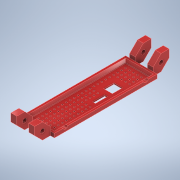
# Autodesk Inventor part: Prod05.3.2 - SKR1.4 Turbo Case Front
Saved by Autodesk Inventor 2021 (Build 250183000, 183)
## iProperties
Created: 2021-06-22
Part Number: Prod05.3.2 - SKR1.4 Turbo Case Front
Material: Generic
Document SubType Name: Modeling
Designer: alexr
Density: 1 g/cm^3
Appearance: Red
Author: alexr
Autodesk Inventor part; units mm, degrees
ref_plane "YZ Plane" through (0, 0, 0) normal (1, 0, 0) x (0, 1, 0)
ref_plane "XZ Plane" through (0, 0, 0) normal (0, 1, 0) x (-1, 0, 0)
ref_plane "XY Plane" through (0, 0, 0) normal (0, 0, 1) x (1, 0, 0)
sketch "Base Profile" plane through (0, 0, 0) normal (1, 0, 0) x (0, 1, 0)
  line L0 (10, 0) -> (20, 0)
  line L1 (20, 0) -> (20, -10)
  line L2 (10, -20) -> (5, -20)
  line L3 (0, -20) -> (0, -10)
  line L4 (0, -20) -> (0, -150)
  line L5 (5, -20) -> (5, -150)
  line L6 (5, -150) -> (10, -150)
  line L7 (20, -160) -> (20, -170)
  line L8 (20, -170) -> (10, -170)
  line L9 (0, -160) -> (0, -150)
  line L10 (0, -160) -> (10, -170)
  line L11 (10, 0) -> (0, -10)
  line L12 (20, -10) -> (10, -20)
  line L13 (10, -150) -> (20, -160)
  point P0 (0, 0)
  point P1 (20, -20)
  point P2 (10, -10)
  point P3 (20, -150)
  point P4 (0, -170)
  point P5 (10, -160)
  dimension "d0" = 20
  dimension "d1" = 20
  dimension "d3" = 130
  dimension "d4" = 5
  dimension "d5" = 20
  dimension "d6" = 20
  constraints: 28 end point, 8 point on line, 5 parallel, 2 horizontal, 2 perpendicular, 1 vertical
  measures "d0" distance of point (20, -20) L3.start
  measures "d1" distance of L0.end point (20, -20)
  measures "d3" distance of L3.start L4.end
  measures "d4" distance between parallel lines of L4 L5
  measures "d5" distance of L7.end point (0, -170)
  measures "d6" distance of point (20, -150) L7.end
extrude "Base Extrusion" add sketch "Base Profile" along normal blind 40
hole "Fixing Holes" at (0, 10, -160) at (0, 10, -10) direction (1, 0, 0) diameter 5.5 end through all
sketch "Cutouts" plane through (0, 0, -160) normal (0, -1, 0) x (1, 0, 0)
  line L0 (0, 10) -> (40, 10) projected
  line L1 (0, 10) -> (5.1, 10)
  line L2 (5.1, 10) -> (5.1, -10)
  line L3 (5.1, -10) -> (0, -10)
  line L4 (0, -10) -> (0, 10)
  line L5 (40, -10) -> (40, 0) projected
  line L6 (40, -10) -> (34.9, -10)
  line L7 (34.9, -10) -> (34.9, 10)
  line L8 (34.9, 10) -> (40, 10)
  line L9 (40, 10) -> (40, -10)
  line L10 (40, 160) -> (40, 150) projected
  line L11 (40, 160) -> (34.9, 160)
  line L12 (34.9, 160) -> (34.9, 140)
  line L13 (34.9, 140) -> (40, 140)
  line L14 (40, 140) -> (40, 160)
  line L15 (0, 160) -> (5.1, 160)
  line L16 (5.1, 160) -> (5.1, 140)
  line L17 (5.1, 140) -> (0, 140)
  line L18 (0, 140) -> (0, 160)
  line L19 (18.75, 43.5) -> (29.75, 43.5)
  line L20 (29.75, 43.5) -> (29.75, 56.5)
  line L21 (29.75, 56.5) -> (18.75, 56.5)
  line L22 (18.75, 56.5) -> (18.75, 43.5)
  line L23 (40, 150) -> (40, 0) projected
  line L24 (0, -10) -> (40, -10) projected
  line L25 (26, 62.5) -> (29.75, 62.5)
  line L26 (29.75, 62.5) -> (29.75, 78)
  line L27 (29.75, 78) -> (26, 78)
  line L28 (26, 78) -> (26, 62.5)
  line L29 (12.4, -10) -> (27.6, -10)
  line L30 (27.6, -10) -> (27.6, 10)
  line L31 (27.6, 10) -> (12.4, 10)
  line L32 (12.4, 10) -> (12.4, -10)
  line L33 (0, 160) -> (40, 160) projected
  line L34 (12.4, 160) -> (27.6, 160)
  line L35 (27.6, 160) -> (27.6, 140)
  line L36 (27.6, 140) -> (12.4, 140)
  line L37 (12.4, 140) -> (12.4, 160)
  line L38 (35, 95) -> (35, 125) construction
  line L39 (5, 125) -> (5, 95) construction
  line L40 (0, 150) -> (0, 0) projected
  point P0 (34.9, 10)
  point P1 (12.4, 10)
  point P2 (27.6, 10)
  point P3 (5, 20)
  point P4 (5, 25)
  point P5 (5, 30)
  point P6 (5, 35)
  point P7 (5, 40)
  point P8 (5, 45)
  point P9 (5, 50)
  point P10 (5, 55)
  point P11 (5, 60)
  point P12 (5, 65)
  point P13 (5, 70)
  point P14 (5, 75)
  point P15 (5, 80)
  point P16 (5, 85)
  point P17 (5, 90)
  point P18 (5, 95)
  point P19 (5, 100)
  point P20 (5, 105)
  point P21 (5, 110)
  point P22 (5, 115)
  point P23 (5, 120)
  point P24 (5, 125)
  point P25 (5, 130)
  point P26 (10, 20)
  point P27 (10, 25)
  point P28 (10, 30)
  point P29 (10, 35)
  point P30 (10, 40)
  point P31 (10, 45)
  point P32 (10, 50)
  point P33 (10, 55)
  point P34 (10, 60)
  point P35 (10, 65)
  point P36 (10, 70)
  point P37 (10, 75)
  point P38 (10, 80)
  point P39 (10, 85)
  point P40 (10, 90)
  point P41 (10, 95)
  point P42 (10, 100)
  point P43 (10, 105)
  point P44 (10, 110)
  point P45 (10, 115)
  point P46 (10, 120)
  point P47 (10, 125)
  point P48 (10, 130)
  point P49 (15, 20)
  point P50 (15, 25)
  point P51 (15, 30)
  point P52 (15, 35)
  point P53 (15, 40)
  point P54 (15, 45)
  point P55 (15, 50)
  point P56 (15, 55)
  point P57 (15, 60)
  point P58 (15, 65)
  point P59 (15, 70)
  point P60 (15, 75)
  point P61 (15, 80)
  point P62 (15, 85)
  point P63 (15, 90)
  point P64 (15, 95)
  point P65 (15, 100)
  point P66 (15, 105)
  point P67 (15, 110)
  point P68 (15, 115)
  point P69 (15, 120)
  point P70 (15, 125)
  point P71 (15, 130)
  point P72 (20, 20)
  point P73 (20, 25)
  point P74 (20, 30)
  point P75 (20, 35)
  point P76 (20, 40)
  point P77 (20, 45)
  point P78 (20, 50)
  point P79 (20, 55)
  point P80 (20, 60)
  point P81 (20, 65)
  point P82 (20, 70)
  point P83 (20, 75)
  point P84 (20, 80)
  point P85 (20, 85)
  point P86 (20, 90)
  point P87 (20, 95)
  point P88 (20, 100)
  point P89 (20, 105)
  point P90 (20, 110)
  point P91 (20, 115)
  point P92 (20, 120)
  point P93 (20, 125)
  point P94 (20, 130)
  point P95 (25, 20)
  point P96 (25, 25)
  point P97 (25, 30)
  point P98 (25, 35)
  point P99 (25, 40)
  point P100 (25, 45)
  point P101 (25, 50)
  point P102 (25, 55)
  point P103 (25, 60)
  point P104 (25, 65)
  point P105 (25, 70)
  point P106 (25, 75)
  point P107 (25, 80)
  point P108 (25, 85)
  point P109 (25, 90)
  point P110 (25, 95)
  point P111 (25, 100)
  point P112 (25, 105)
  point P113 (25, 110)
  point P114 (25, 115)
  point P115 (25, 120)
  point P116 (25, 125)
  point P117 (25, 130)
  point P118 (30, 20)
  point P119 (30, 25)
  point P120 (30, 30)
  point P121 (30, 35)
  point P122 (30, 40)
  point P123 (30, 45)
  point P124 (30, 50)
  point P125 (30, 55)
  point P126 (30, 60)
  point P127 (30, 65)
  point P128 (30, 70)
  point P129 (30, 75)
  point P130 (30, 80)
  point P131 (30, 85)
  point P132 (30, 90)
  point P133 (30, 95)
  point P134 (30, 100)
  point P135 (30, 105)
  point P136 (30, 110)
  point P137 (30, 115)
  point P138 (30, 120)
  point P139 (30, 125)
  point P140 (30, 130)
  point P141 (35, 20)
  point P142 (35, 25)
  point P143 (35, 30)
  point P144 (35, 35)
  point P145 (35, 40)
  point P146 (35, 45)
  point P147 (35, 50)
  point P148 (35, 55)
  point P149 (35, 60)
  point P150 (35, 65)
  point P151 (35, 70)
  point P152 (35, 75)
  point P153 (35, 80)
  point P154 (35, 85)
  point P155 (35, 90)
  point P156 (35, 95)
  point P157 (35, 100)
  point P158 (35, 105)
  point P159 (35, 110)
  point P160 (35, 115)
  point P161 (35, 120)
  point P162 (35, 125)
  point P163 (35, 130)
  dimension "d18" = 5.1
  dimension "d20" = 5.1
  dimension "d21" = 20
  dimension "d22" = 5.1
  dimension "d23" = 20
  dimension "d24" = 5.1
  dimension "d25" = 20
  dimension "d27" = 53.5
  dimension "d33" = 15.5
  dimension "d34" = 6
  dimension "d36" = 15.2
  dimension "d37" = 20
  dimension "d38" = 15.2
  dimension "d39" = 20
  dimension "d40" = 7.3
  dimension "d41" = 7.3
  dimension "d44" = 30
  dimension "d45" = 30
  dimension "d47" = 5
  dimension "d110" = 5
  dimension "d111" = 10.25
  dimension "d112" = 10.25
  dimension "d113" = 14
  dimension "d115" = 82
  dimension "d116" = 0
  dimension "d117" = 10
  dimension "d118" = 0
  dimension "d119" = 150
  dimension "d120" = 0
  dimension "d121" = 160
  dimension "d122" = 35
  dimension "d123" = 5.1
  dimension "d124" = 150
  dimension "d125" = 12.4
  dimension "d126" = 0
  dimension "d127" = 12.4
  dimension "d128" = 150
  dimension "d129" = 12.4
  dimension "d130" = 170
  dimension "d131" = 27.6
  dimension "d132" = 150
  dimension "d133" = 34.9
  dimension "d134" = 150
  dimension "d135" = 65
  dimension "d136" = 11
  dimension "d146" = 5
  dimension "d147" = 10
  dimension "d150" = 5
  dimension "d153" = 5
  constraints: 68 end point, 17 parallel, 9 horizontal, 8 perpendicular, 2 point on line, 1 vertical, 160 other
  measures "d18" distance of L2.end L3.end
  measures "d20" distance of L7.end L8.end
  measures "d21" distance of L6.end L7.end
  measures "d22" distance of L13.end L12.end
  measures "d23" distance of L12.end L11.end
  measures "d24" distance of L16.end L17.end
  measures "d25" distance of L15.end L16.end
  measures "d27" distance between parallel lines of L24 L19
  measures "d33" distance of L26.end L25.end
  measures "d34" distance between parallel lines of L21 L25
  measures "d36" distance of L31.end L30.end
  measures "d37" distance of L30.end L29.end
  measures "d38" distance of L35.end L36.end
  measures "d39" distance of L34.end L35.end
  measures "d40" distance between parallel lines of L12 L35
  measures "d41" distance between parallel lines of L30 L7
  measures "d44" distance of L39.start L38.end
  measures "d45" distance of L38.end L38.start
  measures "d47" distance between parallel lines of L40 L39
  measures "d110" distance between parallel lines of L10 L38
  measures "d111" distance between parallel lines of L10 L26
  measures "d112" distance between parallel lines of L10 L20
  measures "d113" distance between parallel lines of L10 L28
  measures "d115" distance between parallel lines of L27 L33
  measures "d116" distance from line of point (40, 150) L5
  measures "d117" distance from line of point (40, 150) L33
  measures "d118" distance from line of point (40, 10) L5
  measures "d119" distance from line of point (40, 10) L33
  measures "d120" distance from line of point (40, 0) L5
  measures "d121" distance from line of point (40, 0) L33
  measures "d122" distance from line of L38.end L33
  measures "d123" distance from line of point (34.9, 10) L5
  measures "d124" distance from line of point (34.9, 10) L33
  measures "d125" distance from line of point (27.6, 160) L5
  measures "d126" distance from line of point (27.6, 160) L33
  measures "d127" distance from line of point (27.6, 10) L5
  measures "d128" distance from line of point (27.6, 10) L33
  measures "d129" distance from line of point (27.6, -10) L5
  measures "d130" distance from line of point (27.6, -10) L33
  measures "d131" distance from line of point (12.4, 10) L5
  measures "d132" distance from line of point (12.4, 10) L33
  measures "d133" distance from line of point (5.1, 10) L5
  measures "d134" distance from line of point (5.1, 10) L33
  measures "d135" distance from line of L39.end L33
  measures "d136" distance between parallel lines of L20 L22
  measures "d146" distance from line of L40 point (5, 20)
  measures "d147" distance from line of L1 point (5, 20)
  measures "d150" distance of point (5, 20) point (5, 25)
  measures "d153" distance of point (5, 20) point (10, 20)
hole "Vents" at (10, 0, -140) at (30, 0, -140) at (30, 0, -135) at (25, 0, -140) at (25, 0, -135) at (20, 0, -140) at (20, 0, -135) at (15, 0, -140) at (15, 0, -135) at (10, 0, -135) at (10, 0, -130) at (15, 0, -130) at (20, 0, -125) at (25, 0, -125) at (25, 0, -130) at (20, 0, -130) at (30, 0, -130) at (30, 0, -125) at (15, 0, -125) at (10, 0, -125) at (10, 0, -120) at (10, 0, -115) at (10, 0, -110) at (10, 0, -105) at (10, 0, -100) at (10, 0, -95) at (15, 0, -95) at (15, 0, -90) at (15, 0, -85) at (10, 0, -90) at (10, 0, -85) at (20, 0, -95) at (20, 0, -90) at (20, 0, -85) at (20, 0, -80) at (25, 0, -75) at (20, 0, -75) at (30, 0, -75) at (30, 0, -70) at (30, 0, -65) at (30, 0, -60) at (30, 0, -55) at (30, 0, -50) at (30, 0, -45) at (30, 0, -40) at (30, 0, -35) at (30, 0, -30) at (25, 0, -30) at (25, 0, -35) at (20, 0, -35) direction (0, 1, 0) diameter 2 end through all and at (20, 0, -30) (15, 0, -30) (15, 0, -35) (10, 0, -35) (10, 0, -30) (10, 0, -40) (15, 0, -40) (10, 0, -80) (15, 0, -80) (10, 0, -75) (15, 0, -75) (10, 0, -70) (15, 0, -70) (20, 0, -70) (25, 0, -70) (25, 0, -65) (25, 0, -60) (25, 0, -55) (25, 0, -50) (25, 0, -45) (25, 0, -40) (20, 0, -40) (20, 0, -45) (20, 0, -50) (20, 0, -55) (20, 0, -65) (20, 0, -60) (15, 0, -65) (15, 0, -60) (10, 0, -65) (10, 0, -60) (10, 0, -55) (15, 0, -55) (15, 0, -50) (10, 0, -50) (10, 0, -45) (15, 0, -45)
extrude "Cutouts Subtract" cut sketch "Cutouts" against normal blind 40 contours L0 L2 L3 L4 | L18 L15 L16 L17 | L0 L30 L24 L32 | L0 L9 L5 L6 L7 | L33 L35 L36 L37 | L13 L12 L11 L10 L14 | L22 L21 L20 L19 | L28 L27 L26 L25
sketch "Structure" plane through (0, 5, -20) normal (0, 1, 0) x (1, 0, 0)
  line L0 (35, 125) -> (5, 125)
  line L1 (5, 125) -> (5, 5)
  line L2 (5, 5) -> (35, 5)
  line L3 (35, 5) -> (35, 125)
  line L4 (0, 130) -> (0, 0) projected
  line L5 (12.4, 0) -> (27.6, 0) projected
  line L6 (40, 130) -> (40, 0) projected
  line L7 (12.4, 130) -> (27.6, 130) projected
  point P0 (0, -20)
  dimension "d137" = 5
  dimension "d138" = 5
  dimension "d139" = 5
  dimension "d140" = 5
  constraints: 8 end point, 2 parallel, 1 horizontal, 1 perpendicular
  measures "d137" distance between parallel lines of L4 L1
  measures "d138" distance between parallel lines of L5 L2
  measures "d139" distance between parallel lines of L6 L3
  measures "d140" distance between parallel lines of L7 L0
extrude "Structure Subtract" cut sketch "Structure" against normal blind 3.5
chamfer "Structure Clearance" distance 2.5 angle 45 4 edges at (35, 5, -85) (20, 5, -145) (5, 5, -85) (20, 5, -25)
sketch "Standoff Clearance" plane through (40, 0, 0) normal (1, 0, 0) x (0, 0, -1)
  circle A0 centre (34.075, 6) radius 3.25
  line L0 (20, 0) -> (150, 0) projected
  line L1 (0, 10) -> (0, 20) projected
  circle A1 centre (135.925, 6) radius 3.25
  line L2 (170, 20) -> (170, 10) projected
  point P0 (0, 0)
  dimension "d163" = 6.5
  dimension "d164" = 6
  dimension "d165" = 34.075
  dimension "d166" = 6.5
  dimension "d167" = 6
  dimension "d168" = 34.075
  dimension "d171" = 101.85
  constraints: 2 centre point
  measures "d163" diameter of A0
  measures "d164" distance from line of A0.centre L0
  measures "d165" distance from line of L1 A0.centre
  measures "d166" diameter of A1
  measures "d167" distance from line of L0 A1.centre
  measures "d168" distance from line of L2 A1.centre
  measures "d171" distance of A1.centre A0.centre
extrude "Standoff Clearance Subtract" cut sketch "Standoff Clearance" against normal blind 5
equation "\"d165\" = d168"
body "Solid1"
